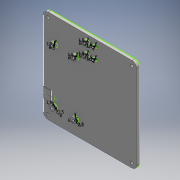
# Autodesk Inventor part: groundplate
Saved by Autodesk Inventor 2016 (Build 200138000, 138)
## iProperties
Created: 2018-12-20
Part Number: groundplate
Material: Generic
Document SubType Name: Modeling
Designer: nerv
Density: 1 g/cm^3
Appearance: Default
Author: nerv
Autodesk Inventor part; units mm, degrees
ref_plane "YZ Plane" through (0, 0, 0) normal (1, 0, 0) x (0, 1, 0)
ref_plane "XZ Plane" through (0, 0, 0) normal (0, 1, 0) x (-1, 0, 0)
ref_plane "XY Plane" through (0, 0, 0) normal (0, 0, 1) x (1, 0, 0)
sketch "Sketch1" plane through (0, 0, 0) normal (0, 1, 0) x (-1, 0, 0)
  line L0 (-12, 95) -> (-12, 5)
  line L1 (-12, 5) -> (-12, 95)
  line L2 (-7, 100) -> (76.1843, 100)
  line L3 (76.1843, 100) -> (-7, 100)
  line L4 (76.0718, 100) -> (83, 100)
  line L5 (-7, 100) -> (83, 100)
  line L6 (88, 11.9282) -> (88, 5)
  line L7 (88, 95) -> (88, 5)
  line L8 (-0.0718, 0) -> (-7, 0)
  line L9 (-7, 0) -> (83, 0)
  arc A0 (-12, 5) -> (-7, 0) centre (-7, 5) ccw
  arc A1 (-7, 100) -> (-12, 95) centre (-7, 95) ccw
  line L10 (88, 5) -> (88, 95)
  arc A2 (88, 95) -> (83, 100) centre (83, 95) ccw
  arc A3 (83, 0) -> (88, 5) centre (83, 5) ccw
  arc A4 (-12, 5) -> (-7, 0) centre (-7, 5) ccw
  circle A5 centre (-7, 5) radius 1.5
  circle A6 centre (-7, 95) radius 1.5
  circle A7 centre (83, 95) radius 1.5
  circle A8 centre (83, 5) radius 1.5
  line L11 (88, 17.761) -> (79.7328, 17.761)
  line L12 (79.7328, 17.761) -> (79.7328, 28.761)
  line L13 (79.7328, 28.761) -> (88, 28.761)
  line L14 (88, 28.761) -> (88, 17.761)
  constraints: 30 end point, 10 point on circle, 9 centre point, 4 coincident, 4 horizontal, 4 tangent, 2 collinear, 2 parallel, 1 perpendicular, 1 vertical
extrude "Extrusion1" add sketch "Sketch1" against normal blind 3 contours A1 L2 L4 A2 L7 L13 L12 L11 L6 A3 L9 L8 A0 L0
extrude "Extrusion2" add sketch "Sketch1" against normal blind 3.2 contours L7 L11 L12 L13
sketch "PiHoles" plane through (0, -3, 0) normal (0, -1, 0) x (1, 0, 0)
  line L0 (-79.7328, 28.761) -> (-79.7328, 17.761) projected
  line L1 (-88, 5) -> (-88, 95) projected
  circle A0 centre (-76, 15.761) radius 1.25
  circle A1 centre (-76, 15.761) radius 3
  circle A2 centre (-76, 73.761) radius 1.25
  circle A3 centre (-76, 73.761) radius 3
  circle A4 centre (-53, 15.761) radius 1.25
  circle A5 centre (-53, 15.761) radius 3
  circle A6 centre (-53, 73.761) radius 1.25
  circle A7 centre (-53, 73.761) radius 3
  circle A8 centre (-53, 73.761) radius 0.75
  circle A9 centre (-53, 15.761) radius 0.75
  circle A10 centre (-76, 73.761) radius 0.75
  circle A11 centre (-76, 15.761) radius 0.75
  circle A12 centre (-41.4372, 81.0897) radius 1.25
  circle A13 centre (-41.4372, 81.0897) radius 3
  circle A14 centre (-41.4372, 81.0897) radius 0.75
  circle A15 centre (-41.4178, 92.9645) radius 0.75
  circle A16 centre (-41.4178, 92.9645) radius 1.25
  circle A17 centre (-41.4178, 92.9645) radius 3
  circle A18 centre (-32.9361, 81.2633) radius 0.75
  circle A19 centre (-32.9361, 81.2633) radius 1.25
  circle A20 centre (-32.9361, 81.2633) radius 2
  circle A21 centre (-32.9166, 93.1381) radius 0.75
  circle A22 centre (-32.9166, 93.1381) radius 1.25
  circle A23 centre (-32.9166, 93.1381) radius 1.75
  point P0 (-79.7328, 23.261)
  point P1 (-88, 23.261)
  point P2 (-76, 23.261)
  point P3 (-76, 23.261)
  point P4 (-52, 74.761)
  point P5 (-41.4372, 93.09)
  point P6 (-40.4372, 94.09)
  dimension "d4" = 2.5
  dimension "d5" = 6
  dimension "d6" = 2.5
  dimension "d7" = 6
  dimension "d8" = 2.5
  dimension "d9" = 6
  dimension "d10" = 2.5
  dimension "d11" = 6
  dimension "d21" = 1.5
  dimension "d22" = 1.5
  dimension "d23" = 1.5
  dimension "d24" = 1.5
  dimension "d30" = 2.5
  dimension "d31" = 6
  dimension "d32" = 1.5
  dimension "d33" = 2.5
  dimension "d34" = 6
  dimension "d35" = 1.5
  dimension "d40" = 2.5
  dimension "d41" = 4
  dimension "d42" = 1.5
  dimension "d43" = 2.5
  dimension "d44" = 3.5
  dimension "d45" = 1.5
  constraints: 30 coincident, 24 centre point, 1 midpoint, 1 point on line
  measures "d4" diameter of A0
  measures "d5" diameter of A1
  measures "d6" diameter of A2
  measures "d7" diameter of A3
  measures "d8" diameter of A4
  measures "d9" diameter of A5
  measures "d10" diameter of A6
  measures "d11" diameter of A7
  measures "d21" diameter of A8
  measures "d22" diameter of A9
  measures "d23" diameter of A10
  measures "d24" diameter of A11
  measures "d30" diameter of A12
  measures "d31" diameter of A13
  measures "d32" diameter of A14
  measures "d33" diameter of A16
  measures "d34" diameter of A17
  measures "d35" diameter of A15
  measures "d40" diameter of A19
  measures "d41" diameter of A20
  measures "d42" diameter of A18
  measures "d43" diameter of A22
  measures "d44" diameter of A23
  measures "d45" diameter of A21
extrude "Extrusion3" add sketch "PiHoles" along normal blind 3 contours A1 | A3 | A5 | A7
extrude "Extrusion4" cut sketch "PiHoles" against normal blind 2 contours A8 | A9 | A10 | A11
extrude "Extrusion5" add sketch "PiHoles" along normal blind 2 contours A13 | A17
extrude "Extrusion6" cut sketch "PiHoles" against normal blind 2 contours A14 | A15
extrude "Extrusion7" add sketch "PiHoles" along normal blind 2 contours A20 | A23
body "Solid1"
